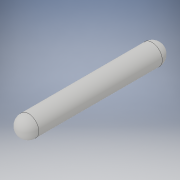
# Autodesk Inventor part: AirTankV1
Saved by Autodesk Inventor 2019 (Build 230136000, 136)
## iProperties
Created: 2021-09-17
Part Number: AirTankV1
Material: Generic
Document SubType Name: Modeling
Designer: timmy
Density: 1 g/cm^3
Appearance: Default
Author: timmy
Autodesk Inventor part; units mm, degrees
ref_plane "YZ Plane" through (0, 0, 0) normal (1, 0, 0) x (0, 1, 0)
ref_plane "XZ Plane" through (0, 0, 0) normal (0, 1, 0) x (-1, 0, 0)
ref_plane "XY Plane" through (0, 0, 0) normal (0, 0, 1) x (1, 0, 0)
sketch "Sketch1" plane through (0, 0, 0) normal (1, 0, 0) x (0, 1, 0)
  line L0 (0, 0) -> (0, -457.2)
  arc A0 (0, -457.2) -> (38.1, -495.3) centre (38.1, -457.2) ccw
  line L1 (38.1, 40.3659) -> (38.1, -495.3)
  arc A1 (38.1, 40.3659) -> (0, 0) centre (38.1, 2.2023) ccw
  dimension "d0" = 457.2
  constraints: 4 end point, 4 point on circle, 3 coincident, 2 centre point, 1 tangent, 1 vertical
  measures "d0" distance of L0.start L0.end
revolve "Revolution1" add sketch "Sketch1" angle 360 about axis through (0, 38.1, 40.3659) along (0, 0, -1)
body "Solid1"
